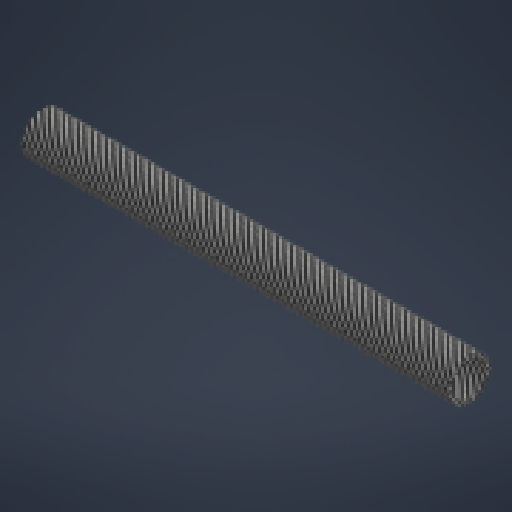
# Autodesk Inventor part: P_Carbon_Pipe_Back
Saved by Autodesk Inventor 2026 (Build 300175000, 175)
## iProperties
Created: 2025-08-24
Part Number: P_Carbon_Pipe_Back
Material: Generisch
Document SubType Name: Modeling
Designer: FAL
Density: 1.55 g/cm^3
Appearance: Vorgabe
Mass: 29.2168 g
Surface Area: 191.009 cm^2
Volume: 18.8496 cm^3
Author: FAL
Autodesk Inventor part; units mm, degrees
ref_plane "YZ Plane" through (0, 0, 0) normal (1, 0, 0) x (0, 1, 0)
ref_plane "XZ Plane" through (0, 0, 0) normal (0, 1, 0) x (-1, 0, 0)
ref_plane "XY Plane" through (0, 0, 0) normal (0, 0, 1) x (1, 0, 0)
sketch "Skizze1" plane through (0, 0, 0) normal (1, 0, 0) x (0, 1, 0)
  circle A0 centre (0, 0) radius 11
  circle A1 centre (0, 0) radius 9
  dimension "d0" = 22
  dimension "d1" = 2
  constraints: 2 centre point, 2 coincident
  measures "d0" diameter of A0
  measures "d1" radial gap between concentric circles of A0 A1
extrude "Extrusion1" add sketch "Skizze1" along normal blind 225
